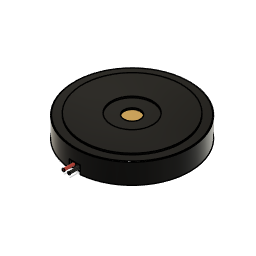
Module Piezzo (Autodesk Fusion 360 design; units mm, degrees)
Autodesk Fusion 360 part; units mm, degrees
sketch "Sketch1" plane through (0, 0, 0) normal (0, 1, 0) x (1, 0, 0)
  circle A0 centre (0, 0) radius 10.5
  dimension "d1" = 21
  constraint coincident A0.centre origin
  measures "d1" diameter of A0
extrude "Extrude1" add sketch "Sketch1" along normal blind 4
sketch "Sketch2" plane through (0, 4, 0) normal (0, 1, 0) x (-1, 0, 0)
  circle A0 centre (0, 0) radius 10.5
  circle A1 centre (0, 0) radius 1.5
  dimension "d4" = 3
  constraint coincident A0.centre A1.centre
  measures "d4" diameter of A1
extrude "Extrude2" cut sketch "Sketch2" against normal blind 0.5 contours A1
sketch "Sketch3" plane through (0, 4, 0) normal (0, 1, 0) x (-1, 0, 0)
  circle A0 centre (0, 0) radius 1.5
  circle A1 centre (0, 0) radius 10.5
  circle A2 centre (0, 0) radius 9
  circle A3 centre (0, 0) radius 3.75
  dimension "d7" = 1.5
  dimension "d20" = 7.5
  constraint coincident A0.centre A1.centre
  measures "d20" diameter of A3
extrude "Extrude3" cut sketch "Sketch3" against normal blind 0.25
fillet "Fillet1" radius 0.1 1 edges at (-9.7894, 3.75, -3.797)
ref_plane "WorkPlane1" through (0, 0, 10.5) normal (0, 0, 1) x (1, 0, 0)
sketch "Sketch4" plane through (0, 0, 10.5) normal (0, 0, 1) x (1, 0, 0)
  line L0 (-1, 0) -> (1, 0)
  line L1 (1, 0) -> (1, 1.5)
  line L2 (1, 1.5) -> (-1, 1.5)
  line L3 (-1, 1.5) -> (-1, 0)
  line L4 (10.5, 0) -> (-10.5, 0)
  dimension "d12" = 1.5
  dimension "d13" = 2
  constraint horizontal L0
  constraint vertical L1
  constraint horizontal L2
  constraint vertical L3
  constraint coincident L0.start L4
  constraint midpoint origin L0
  measures "d12" distance of L0.start L2.end
  measures "d13" distance of L1 L3
extrude "Extrude4" cut sketch "Sketch4" against normal blind 0.5
sketch "Sketch5" plane through (0, 0, 10) normal (0, 0, 1) x (1, 0, 0)
  line L0 (1, 0) -> (1, 1.5)
  line L1 (1, 1.5) -> (-1, 1.5)
  line L2 (-1, 1.5) -> (-1, 0)
  line L3 (-1, 0) -> (1, 0)
  line L4 (9, 4) -> (-9, 4)
  line L5 (0, 1.5) -> (0, 0) construction
  line L6 (0, 0.75) -> (-1, 0.75) construction
  circle A0 centre (-0.5, 0.75) radius 0.25
  circle A1 centre (0.5, 0.75) radius 0.25
  dimension "d16" = 0.5
  constraint coincident L5.end origin
  constraint midpoint L1 L5.start
  constraint coincident L2 L6.end
  constraint midpoint L2 L6.end
  constraint coincident L6 A0.centre
  constraint horizontal L6
  constraint midpoint L5 L6.start
  constraint midpoint L6 A0.centre
  constraint symmetric L5 A0 A1
  measures "d16" diameter of A0
extrude "Extrude5" add sketch "Sketch5" along normal blind 2 contours A0 | A1
